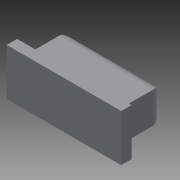
# Autodesk Inventor part: PRZYCISK
Saved by Autodesk Inventor 2014 (Build 180170000, 170)
## iProperties
Created: 2017-04-20
Part Number: PRZYCISK
Material: Ogólny
Document SubType Name: Modeling
Designer: hpdc7700
Density: 1 g/cm^3
Appearance: Domyślna
Author: hpdc7700
Autodesk Inventor part; units mm, degrees
ref_plane "YZ Plane" through (0, 0, 0) normal (1, 0, 0) x (0, 1, 0)
ref_plane "XZ Plane" through (0, 0, 0) normal (0, 1, 0) x (-1, 0, 0)
ref_plane "XY Plane" through (0, 0, 0) normal (0, 0, 1) x (1, 0, 0)
sketch "Szkic1" plane through (0, 0, 0) normal (0, 1, 0) x (-1, 0, 0)
  line L0 (-4.5, -1.5) -> (4.5, -1.5)
  line L1 (4.5, -1.5) -> (4.5, 1.5)
  line L2 (4.5, 1.5) -> (-4.5, 1.5)
  line L3 (-4.5, 1.5) -> (-4.5, -1.5)
  line L4 (-4.5, -1.5) -> (4.5, 1.5) construction
  line L5 (4.5, -1.5) -> (-4.5, 1.5) construction
  point P0 (0, 0)
  dimension "d0" = 9
  dimension "d1" = 3
  constraints: 12 end point, 2 midpoint, 2 parallel, 1 horizontal, 1 perpendicular
  measures "d0" distance of L2.end L1.end
  measures "d1" distance of L1.end L0.end
extrude "Wyciągnięcie proste1" add sketch "Szkic1" along normal blind 4
sketch "Szkic2" plane through (0, 0, 0) normal (0, -1, 0) x (1, 0, 0)
  line L0 (-5.5, -2.25) -> (5.5, -2.25)
  line L1 (5.5, -2.25) -> (5.5, 2.25)
  line L2 (5.5, 2.25) -> (-5.5, 2.25)
  line L3 (-5.5, 2.25) -> (-5.5, -2.25)
  line L4 (-5.5, -2.25) -> (5.5, 2.25) construction
  line L5 (5.5, -2.25) -> (-5.5, 2.25) construction
  point P0 (0, 0)
  dimension "d4" = 11
  dimension "d5" = 4.5
  constraints: 12 end point, 2 midpoint, 2 parallel, 1 horizontal, 1 perpendicular
  measures "d4" distance of L2.end L1.end
  measures "d5" distance of L1.end L0.end
extrude "Wyciągnięcie proste2" add sketch "Szkic2" along normal blind 1
fillet "Zaokrąglenie1" radius 1 4 edges at (0, 4, 1.5) (-4.5, 4, 0) (0, 4, -1.5) (4.5, 4, 0)
